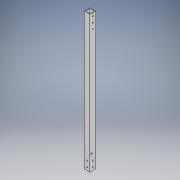
# Autodesk Inventor part: 25in 1x1 Beam
Saved by Autodesk Inventor 2018 (Build 220112000, 112)
## iProperties
Created: 2019-01-16
Part Number: 25in 1x1 Beam
Material: Generic
Document SubType Name: Modeling
Designer: Gabriel
Density: 1 g/cm^3
Appearance: Default
Author: Gabriel
Autodesk Inventor part; units mm, degrees
ref_plane "YZ Plane" through (0, 0, 0) normal (1, 0, 0) x (0, 1, 0)
ref_plane "XZ Plane" through (0, 0, 0) normal (0, 1, 0) x (-1, 0, 0)
ref_plane "XY Plane" through (0, 0, 0) normal (0, 0, 1) x (1, 0, 0)
sketch "Sketch1" plane through (0, 0, 0) normal (0, 1, 0) x (-1, 0, 0)
  line L0 (1.8436, -2.4426) -> (-23.5564, -2.4426)
  line L1 (-23.5564, -2.4426) -> (-23.5564, 22.9574)
  line L2 (-23.5564, 22.9574) -> (1.8436, 22.9574)
  line L3 (1.8436, 22.9574) -> (1.8436, -2.4426)
  line L4 (-20.3814, 0.7324) -> (-1.3314, 0.7324)
  line L5 (-1.3314, 0.7324) -> (-1.3314, 19.7824)
  line L6 (-1.3314, 19.7824) -> (-20.3814, 19.7824)
  line L7 (-20.3814, 19.7824) -> (-20.3814, 0.7324)
  point P0 (0, 0)
  dimension "d0" = 25.4
  dimension "d1" = 25.4
  dimension "d2" = 3.175
  constraints: 16 end point, 4 parallel, 2 perpendicular, 1 horizontal, 3 other
  measures "d0" distance of L1.end L2.end
  measures "d1" distance of L0.end L1.end
  measures "d2" distance between parallel lines of L0 L4
extrude "Extrusion1" add sketch "Sketch1" along normal blind 609.6
sketch "Sketch2" plane through (-1.8436, 0, -2.4426) normal (-1, 0, 0) x (0, 0, 1)
  line L0 (22.225, 0) -> (3.175, 0) construction
  line L1 (12.7, 0) -> (12.7, 12.7) construction
  line L2 (12.7, 12.7) -> (12.7, 38.1) construction
  line L3 (3.175, 609.6) -> (22.225, 609.6) construction
  line L4 (12.7, 609.6) -> (12.7, 596.9) construction
  line L5 (12.7, 596.9) -> (12.7, 571.5) construction
  circle A0 centre (12.7, 596.9) radius 2.5797
  circle A1 centre (12.7, 571.5) radius 2.5797
  circle A2 centre (12.7, 12.7) radius 2.5797
  circle A3 centre (12.7, 38.1) radius 2.5797
  point P0 (2.4426, 0)
  dimension "d5" = 12.7
  dimension "d6" = 25.4
  dimension "d7" = 12.7
  dimension "d8" = 25.4
  dimension "d9" = 5.1594
  dimension "d10" = 5.1594
  dimension "d11" = 5.1594
  dimension "d12" = 5.1594
  constraints: 8 end point, 4 centre point, 4 coincident, 2 midpoint, 2 point on line, 2 vertical
  measures "d5" distance of L1.start L1.end
  measures "d6" distance of L1.end L2.end
  measures "d7" distance of L4.start L4.end
  measures "d8" distance of L4.end L5.end
  measures "d9" diameter of A0
  measures "d10" diameter of A1
  measures "d11" diameter of A2
  measures "d12" diameter of A3
extrude "Extrusion2" cut sketch "Sketch2" against normal blind 635
sketch "Sketch3" plane through (-1.8436, 0, -2.4426) normal (-1, 0, 0) x (0, 0, 1)
  circle A0 centre (12.7, 571.5) radius 2.5797 construction
  line L0 (12.7, 571.5) -> (12.7, 546.1) construction
  circle A1 centre (12.7, 546.1) radius 2.5797
  point P0 (2.4426, 0)
  dimension "d15" = 25.4
  dimension "d16" = 5.1594
  constraints: 2 end point, 1 centre point, 1 coincident, 1 vertical
  measures "d15" distance of L0.start L0.end
  measures "d16" diameter of A1
extrude "Extrusion3" cut sketch "Sketch3" against normal blind 127
sketch "Sketch4" plane through (-1.8436, 0, 22.9574) normal (0, 0, 1) x (1, 0, 0)
  line L0 (0, 0) -> (25.4, 0) construction
  line L1 (12.7, 0) -> (12.7, 12.7) construction
  line L2 (12.7, 12.7) -> (12.7, 38.1) construction
  circle A0 centre (12.7, 12.7) radius 2.5797
  circle A1 centre (12.7, 38.1) radius 2.5797
  point P0 (1.8436, 0)
  dimension "d19" = 12.7
  dimension "d20" = 25.4
  dimension "d21" = 5.1594
  dimension "d22" = 5.1594
  constraints: 4 end point, 2 centre point, 2 coincident, 2 vertical, 1 midpoint
  measures "d19" distance of L1.start L1.end
  measures "d20" distance of L1.end L2.end
  measures "d21" diameter of A0
  measures "d22" diameter of A1
extrude "Extrusion4" cut sketch "Sketch4" against normal blind 127
sketch "Sketch5" plane through (23.5564, 0, 22.9574) normal (1, 0, 0) x (0, 0, -1)
  line L0 (0, 0) -> (25.4, 0) construction
  line L1 (0, 0) -> (9.7028, 0) construction
  line L2 (9.7028, 0) -> (9.7028, 68.0974) construction
  circle A0 centre (9.7028, 68.0974) radius 3.302
  point P0 (22.9574, 0)
  dimension "d25" = 9.7028
  dimension "d26" = 68.0974
  dimension "d27" = 6.604
  constraints: 4 end point, 1 centre point, 1 coincident, 1 perpendicular, 1 point on line
  measures "d25" distance of L0.start L1.end
  measures "d26" distance of L1.end L2.end
  measures "d27" diameter of A0
extrude "Extrusion5" cut sketch "Sketch5" against normal blind 50.8
body "Solid1"
